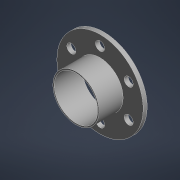
# Autodesk Inventor part: P026-Butée_carter_arbre
Saved by Autodesk Inventor 2021.3 (Build 253353000, 353)
## iProperties
Created: 2022-06-11
Part Number: P026-Butée_carter_arbre
Material: Aluminium
Document SubType Name: Modeling
Designer: Rémi Heredero
Density: 2.7 g/cm^3
Appearance: Par défaut
Author: Rémi Heredero
Autodesk Inventor part; units mm, degrees
ref_plane "YZ Plane" through (0, 0, 0) normal (1, 0, 0) x (0, 1, 0)
ref_plane "XZ Plane" through (0, 0, 0) normal (0, 1, 0) x (-1, 0, 0)
ref_plane "XY Plane" through (0, 0, 0) normal (0, 0, 1) x (1, 0, 0)
sketch "Sketch2" plane through (0, 0, 0) normal (1, 0, 0) x (0, 1, 0)
  line L0 (-2.8, 0) -> (16.8, 0) projected
  line L1 (0, 10.85) -> (0, 11.5)
  line L2 (0, 11.5) -> (12, 11.5)
  line L3 (12, 11.5) -> (12, 21.5)
  line L4 (12, 21.5) -> (14, 21.5)
  line L5 (14, 21.5) -> (14, 10.85)
  line L6 (14, 10.85) -> (0, 10.85)
  point P0 (0, 0)
  point P1 (0, 11.175)
  dimension "d0" = 43
  dimension "d1" = 23
  dimension "d2" = 2
  dimension "d3" = 12
  dimension "d4" = 21.7
  constraints: 12 end point, 5 perpendicular, 1 midpoint, 1 vertical, 1 vertical alignment
  measures "d0" diameter of L4 L0
  measures "d1" diameter of L2 L0
  measures "d2" distance of L3.end L4.end
  measures "d3" distance of L1.end L2.end
  measures "d4" diameter of L6 L0
revolve "Revolution1" add sketch "Sketch2" angle 360 about axis through (0, -10, 0) along (0, 1, 0)
sketch "Sketch4" plane through (0, 14, 0) normal (0, 1, 0) x (1, 0, 0)
  circle A0 centre (0, 0) radius 21.5 construction
  circle A1 centre (0, 0) radius 10.85 construction
  circle A2 centre (0, 0) radius 16.5 construction
  line L0 (14.2894, 8.25) -> (-14.2894, -8.25) construction
  line L1 (-14.2894, 8.25) -> (14.2894, -8.25) construction
  point P0 (0, 16.5)
  point P1 (0, -16.5)
  point P2 (0, 16.5)
  point P3 (0, -16.5)
  dimension "d15" = 33
  dimension "d16" = 60
  dimension "d17" = 60
  constraints: 7 coincident, 6 point on circle, 4 end point, 3 midpoint, 2 vertical alignment, 1 centre point
  measures "d15" diameter of A2
hole "Hole1" at (0, 14, -16.5) at (0, 14, 16.5) at (14.2894, 14, -8.25) at (-14.2894, 14, -8.25) at (14.2894, 14, 8.25) at (-14.2894, 14, 8.25) direction (0, -1, 0) diameter 4.5 end through all clearance for "Flat Head Machine Screw" size "M4" standard "Ansi Metric M Profile"
body "Solid1"
